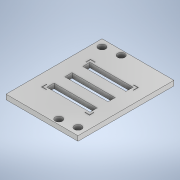
# Autodesk Inventor part: Maska
Saved by Autodesk Inventor 2021 (Build 250183000, 183)
## iProperties
Created: 2021-04-28
Part Number: Maska
Material: Aluminium 6061
Document SubType Name: Modeling
Designer: DESKTOP-12
Density: 2.7 g/cm^3
Appearance: Aluminium — polerowane
Author: DESKTOP-12
Autodesk Inventor part; units mm, degrees
ref_plane "YZ Plane" through (0, 0, 0) normal (1, 0, 0) x (0, 1, 0)
ref_plane "XZ Plane" through (0, 0, 0) normal (0, 1, 0) x (-1, 0, 0)
ref_plane "XY Plane" through (0, 0, 0) normal (0, 0, 1) x (1, 0, 0)
sketch "Szkic1" plane through (0, 0, 0) normal (0, 1, 0) x (-1, 0, 0)
  line L0 (0, 0) -> (30, 0)
  line L1 (30, 0) -> (30, -40)
  line L2 (25, -12) -> (25, -10)
  line L3 (25, -12) -> (25.2, -12)
  line L4 (25.2, -12) -> (25.2, -10)
  line L5 (25.2, -10) -> (25, -10)
  line L6 (24.8, -10.2) -> (24.8, -10)
  line L7 (0, 0) -> (0, -40)
  line L8 (30, -40) -> (0, -40)
  line L9 (24, -11) -> (6, -11)
  line L10 (6, -11) -> (6, -14)
  line L11 (6, -14) -> (24, -14)
  line L12 (24, -14) -> (24, -11)
  line L13 (24, -18.5) -> (6, -18.5)
  line L14 (6, -18.5) -> (6, -21.5)
  line L15 (6, -21.5) -> (24, -21.5)
  line L16 (24, -21.5) -> (24, -18.5)
  line L17 (24, -26) -> (6, -26)
  line L18 (6, -26) -> (6, -29)
  line L19 (6, -29) -> (24, -29)
  line L20 (24, -29) -> (24, -26)
  circle A0 centre (27, -37) radius 1.5
  circle A1 centre (20, -38) radius 1.5
  circle A2 centre (3, -3) radius 1.5
  circle A3 centre (10, -2) radius 1.5
  line L21 (24.8, -10) -> (23.3, -10)
  line L22 (23.3, -10) -> (23.3, -10.2)
  line L23 (23.3, -10.2) -> (24.8, -10.2)
  line L24 (7, -9.8) -> (5, -9.8)
  line L25 (5, -9.8) -> (5, -10)
  line L26 (7, -10) -> (5, -10)
  line L27 (7, -10) -> (7, -9.8)
  line L28 (5.2, -11.7) -> (5.2, -10.2)
  line L29 (5, -10.2) -> (5, -11.7)
  line L30 (5.2, -10.2) -> (5, -10.2)
  line L31 (5, -11.7) -> (5.2, -11.7)
  line L32 (4.8, -28) -> (4.8, -30)
  line L33 (4.8, -30) -> (5, -30)
  line L34 (5, -28) -> (5, -30)
  line L35 (5, -28) -> (4.8, -28)
  line L36 (6.7, -29.8) -> (5.2, -29.8)
  line L37 (5.2, -30) -> (6.7, -30)
  line L38 (5.2, -29.8) -> (5.2, -30)
  line L39 (6.7, -30) -> (6.7, -29.8)
  line L40 (23, -30.2) -> (25, -30.2)
  line L41 (25, -30.2) -> (25, -30)
  line L42 (23, -30) -> (25, -30)
  line L43 (23, -30) -> (23, -30.2)
  line L44 (24.8, -28.3) -> (24.8, -29.8)
  line L45 (25, -29.8) -> (25, -28.3)
  line L46 (24.8, -29.8) -> (25, -29.8)
  line L47 (25, -28.3) -> (24.8, -28.3)
  point P0 (15, -20)
  dimension "d0" = 30
  dimension "d1" = 40
  dimension "d13" = 2
  dimension "d14" = 0.2
  dimension "d15" = 0.2
  dimension "d37" = 18
  dimension "d38" = 3
  dimension "d39" = 6
  dimension "d40" = 11
  dimension "d41" = 6
  dimension "d42" = 18
  dimension "d43" = 3
  dimension "d44" = 18
  dimension "d45" = 3
  dimension "d46" = 4.5
  dimension "d47" = 4.5
  dimension "d48" = 11
  dimension "d49" = 6
  dimension "d50" = 6
  dimension "d51" = 3
  dimension "d52" = 3
  dimension "d53" = 2
  dimension "d54" = 10
  dimension "d55" = 3
  dimension "d56" = 3
  dimension "d57" = 20
  dimension "d58" = 15
  dimension "d61" = 360
  dimension "d65" = 1
  dimension "d66" = 1.5
  dimension "d67" = 0.2
  dimension "d70" = 360
  constraints: 96 end point, 9 perpendicular, 6 horizontal, 6 parallel, 4 centre point, 2 coincident, 1 vertical, 74 other
  measures "d0" distance of L0.start L0.end
  measures "d1" distance of L0.end L1.end
  measures "d13" distance of L2.start L2.end
  measures "d14" distance of L2.start L3.end
  measures "d15" distance of L2.end L6.end
  measures "d37" distance of L11.end L10.end
  measures "d38" distance of L10.end L9.end
  measures "d39" distance from line of L1 L9.start
  measures "d40" distance from line of L0 L9.start
  measures "d41" distance from line of L7 L9.end
  measures "d42" distance of L16.start L15.start
  measures "d43" distance of L15.start L13.end
  measures "d44" distance of L20.start L19.start
  measures "d45" distance of L19.start L17.end
  measures "d46" distance of L16.end L11.end
  measures "d47" distance of L20.end L16.start
  measures "d48" distance from line of L8 L20.start
  measures "d49" distance between parallel lines of L1 L16
  measures "d50" distance between parallel lines of L1 L20
  measures "d51" distance from line of L8 point (27, -37)
  measures "d52" distance from line of L1 point (27, -37)
  measures "d53" distance from line of L8 point (20, -38)
  measures "d54" distance from line of L1 point (20, -38)
  measures "d55" diameter of A0
  measures "d56" diameter of A1
  measures "d57" distance from line of L0 point (15, -20)
  measures "d58" distance from line of L7 point (15, -20)
  measures "d65" distance from line of L12 L2.start
  measures "d66" distance of L6.end L21.end
  measures "d67" distance of L22.end L21.end
extrude "Wyciągnięcie proste2" add sketch "Szkic1" along normal blind 2
